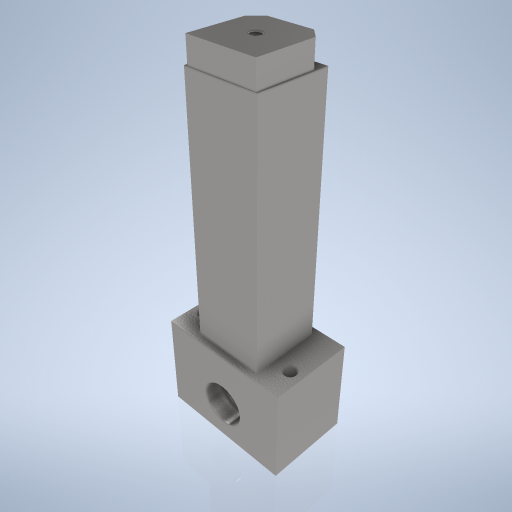
# Autodesk Inventor part: Lagerbock
Saved by Autodesk Inventor 2024.2 (Build 282272000, 272)
## iProperties
Created: 2024-04-02
Part Number: Lagerbock
Material: Stahl, galvanisiert
Document SubType Name: Modeling
Designer: ffogue
Density: 7.85 g/cm^3
Appearance: Galvanisiert
Author: ffogue
Autodesk Inventor part; units mm, degrees
note: some values were not read from the file. Chosen so that the rebuilt part matches the saved one: direction of "Bohrung3".
ref_plane "YZ Plane" through (0, 0, 0) normal (1, 0, 0) x (0, 1, 0)
ref_plane "XZ Plane" through (0, 0, 0) normal (0, 1, 0) x (-1, 0, 0)
ref_plane "XY Plane" through (0, 0, 0) normal (0, 0, 1) x (1, 0, 0)
sketch "Skizze1" plane through (0, 0, 0) normal (0, 0, 1) x (1, 0, 0)
  line L0 (15, -9.5) -> (-15, -9.5)
  line L1 (-15, -9.5) -> (-15, 9.5)
  line L2 (-15, 9.5) -> (15, 9.5)
  line L3 (15, 9.5) -> (15, -9.5)
  line L4 (15, -9.5) -> (-15, 9.5) construction
  line L5 (-15, -9.5) -> (15, 9.5) construction
  point P0 (0, 0)
  dimension "d0" = 30
  dimension "d1" = 19
  constraints: 12 end point, 2 midpoint, 2 parallel, 1 horizontal, 1 perpendicular
  measures "d0" distance of L1.end L2.end
  measures "d1" distance of L0.end L1.end
extrude "Extrusion1" add sketch "Skizze1" along normal blind 22
sketch "Skizze7" plane through (0, 0, 22) normal (0, 0, 1) x (1, 0, 0)
  line L0 (-7.5, -7.5) -> (-7.5, 7.5)
  line L1 (-7.5, 7.5) -> (7.5, 7.5)
  line L2 (7.5, 7.5) -> (7.5, -7.5)
  line L3 (7.5, -7.5) -> (-7.5, -7.5)
  line L4 (15, -9.5) -> (15, 9.5) projected
  point P0 (0, 0)
  point P1 (0, -7.5)
  point P2 (7.5, 0)
  point P3 (15, 0)
  dimension "d36" = 15
  dimension "d37" = 15
  constraints: 8 end point, 3 midpoint, 3 perpendicular, 1 horizontal alignment, 1 vertical, 1 vertical alignment
  measures "d36" distance between parallel lines of L3 L1
  measures "d37" distance between parallel lines of L2 L0
extrude "Extrusion3" add sketch "Skizze7" along normal blind 60
chamfer "Fasen1" distance 2.5 angle 45 2 edges at (-7.5, 7.5, 52) (7.5, 7.5, 52)
sketch "Skizze2" plane through (-15, -9.5, 22) normal (0, 0, 1) x (1, 0, 0)
  line L0 (7, 17.25) -> (23, 17.25)
  line L1 (23, 17.25) -> (23, 1.75)
  line L2 (23, 1.75) -> (7, 1.75)
  line L3 (7, 1.75) -> (7, 17.25)
  line L4 (0, 0) -> (30, 0) projected
  point P0 (15, 9.5)
  point P1 (15, 1.75)
  point P2 (15, 0)
  point P3 (7, 9.5)
  dimension "d4" = 16
  dimension "d7" = 15.5
  constraints: 8 end point, 2 midpoint, 2 parallel, 1 horizontal, 1 horizontal alignment, 1 perpendicular, 1 vertical alignment, 2 other
  measures "d4" distance between parallel lines of L1 L3
  measures "d7" distance between parallel lines of L2 L0
extrude "Extrusion2" add sketch "Skizze2" along normal blind 55
sketch "Skizze3" plane through (-15, -9.5, 82) normal (0, 0, 1) x (1, 0, 0)
  line L0 (23, 1.75) -> (23, 17.25) projected
  line L1 (23, 17.25) -> (7, 17.25) projected
  point P0 (15, 9.5)
  point P1 (15, 9.5)
  point P2 (23, 9.5)
  point P3 (15, 17.25)
  constraints: 2 midpoint, 1 horizontal alignment, 1 vertical alignment
hole "Bohrung1" at (0, 0, 82) direction (0, 0, -1) diameter 2.459 depth 15 tip angle 118 thread size "M3x0.5" class "6H" standard "ISO Metric profile"
sketch "Skizze4" plane through (-15, -9.5, 0) normal (0, -1, 0) x (1, 0, 0)
  line L0 (0, 0) -> (30, 0) projected
  line L1 (7, 77) -> (23, 77) projected
  line L2 (7.5, 82) -> (22.5, 82) projected
  point P0 (15, 0)
  point P1 (15, 9)
  point P2 (15, 0)
  dimension "d43" = 73
  constraints: 1 midpoint, 1 vertical alignment
  measures "d43" distance from line of L2 point (15, 9)
hole "Bohrung2" at (0, -9.5, 9) direction (0, 1, 0) diameter 7.5 depth 9.5 counterbore diameter 10 counterbore depth 4
mirror "Spiegeln1" about plane through (0, 0, 0) normal (0, 1, 0) of "Bohrung2"
sketch "Skizze5" plane through (0, 0, 22) normal (0, 0, 1) x (1, 0, 0)
  circle A0 centre (0, 0) radius 1.2295 projected
  line L0 (15, 9.5) -> (-15, 9.5) projected
  line L1 (-15, -9.5) -> (15, -9.5) projected
  point P0 (12, -3)
  point P1 (-12, -3)
  dimension "d30" = 24
  dimension "d31" = 12
  dimension "d34" = 6.5
  dimension "d35" = 6.5
  measures "d30" distance of point (-12, -3) point (12, -3)
  measures "d31" horizontal distance of point (12, -3) point (0, 0)
  measures "d34" distance from line of L1 point (12, -3)
  measures "d35" distance from line of L1 point (-12, -3)
hole "Bohrung3" at (12, -3, 22) at (-12, -3, 22) direction (0, 0, -1) diameter 3.1 depth 22
